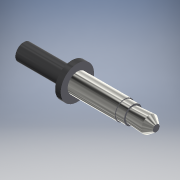
# Autodesk Inventor part: 3,5mm jack
Saved by Autodesk Inventor 2018 (Build 220112000, 112)
## iProperties
Created: 2018-12-13
Part Number: 3,5mm jack
Material: Generic
Document SubType Name: Modeling
Designer: petal
Density: 1 g/cm^3
Appearance: Default
Author: petal
Autodesk Inventor part; units mm, degrees
ref_plane "YZ Plane" through (0, 0, 0) normal (1, 0, 0) x (0, 1, 0)
ref_plane "XZ Plane" through (0, 0, 0) normal (0, 1, 0) x (-1, 0, 0)
ref_plane "XY Plane" through (0, 0, 0) normal (0, 0, 1) x (1, 0, 0)
sketch "Sketch1" plane through (0, 0, 0) normal (0, 0, 1) x (1, 0, 0)
  line L0 (0, 0) -> (0, 3)
  line L1 (0, 3) -> (1, 3)
  line L2 (1, 3) -> (1, 1.75)
  line L3 (0, 0) -> (14, 0)
  line L4 (1, 1.75) -> (9.5, 1.75)
  line L5 (9.5, 1.75) -> (9.5, 1.6)
  line L6 (9.5, 1.6) -> (11, 1.6)
  line L7 (11, 1.6) -> (11, 1.3)
  line L8 (11, 1.3) -> (14, 1.5)
  line L9 (14, 1.5) -> (15.2, 0.6)
  line L10 (15.2, 0.6) -> (15.2, 0)
  line L11 (0, 1.5) -> (-8.6528, 1.5)
  line L12 (-8.6528, 1.5) -> (-8.6528, 0)
  line L13 (0, 0) -> (-8.6528, 0)
  line L14 (14, 0) -> (15.2, 0)
  dimension "d1" = 1
  dimension "d3" = 14
  dimension "d5" = 6
  dimension "d6" = 3.5
  dimension "d7" = 3.2
  dimension "d8" = 2.6
  dimension "d9" = 3
  dimension "d11" = 14
  dimension "d12" = 11
  dimension "d13" = 9.5
  dimension "d15" = 1.2
  dimension "d16" = 1.2
  dimension "d17" = 8.6528
  constraints: 30 end point, 5 horizontal, 4 perpendicular, 3 vertical, 1 midpoint, 1 parallel
  measures "d1" distance of L0.end L1.end
  measures "d3" distance of L0.start L3.end
  measures "d5" diameter of L1 L3
  measures "d6" diameter of L4 L3
  measures "d7" diameter of L6 L3
  measures "d8" diameter of L7.end L3
  measures "d9" diameter of L8.end L3
  measures "d11" horizontal distance of L8.end L0.end
  measures "d12" horizontal distance of L0.end L6.end
  measures "d13" horizontal distance of L0.end L4.end
  measures "d15" horizontal distance of L9.end L3.end
  measures "d16" diameter of L9.end L3
  measures "d17" distance of L11.end L11.start
revolve "Revolution1" add sketch "Sketch1" angle 360 about axis through (0, 0, 0) along (1, 0, 0)
body "Solid1"
